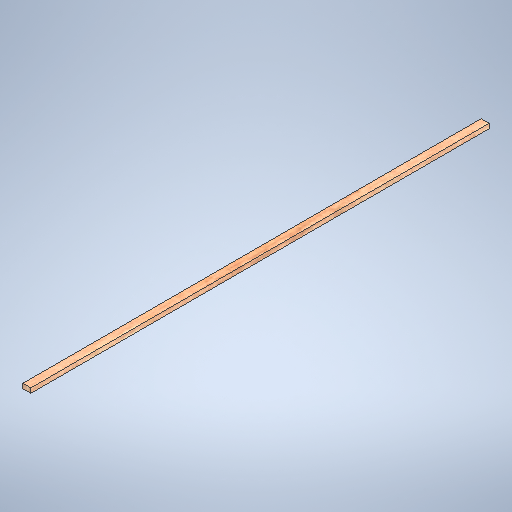
# Autodesk Inventor part: 2P.03.01.14.IM.AilTopSpanBeam
Saved by Autodesk Inventor 2025.2 (Build 292293000, 293)
## iProperties
Created: 2025-01-08
Part Number: 2P.03.01.14.IM.AilTopSpanBeam
Material: Wood (Birch)
Document SubType Name: Modeling
Designer: Imist
Density: 0.55 g/cm^3
Appearance: Birch - Natural Polished
Author: Imist
Autodesk Inventor part; units mm, degrees
ref_plane "YZ Plane" through (0, 0, 0) normal (1, 0, 0) x (0, 1, 0)
ref_plane "XZ Plane" through (0, 0, 0) normal (0, 1, 0) x (-1, 0, 0)
ref_plane "XY Plane" through (0, 0, 0) normal (0, 0, 1) x (1, 0, 0)
sketch "Sketch1" plane through (0, 0, 0) normal (0, 0, 1) x (1, 0, 0)
  line L0 (-2.548, 1.5) -> (2.548, 1.5)
  line L1 (2.548, 1.5) -> (2.548, -1.5)
  line L2 (2.548, -1.5) -> (-2.548, -1.5)
  line L3 (-2.548, -1.5) -> (-2.548, 1.5)
  line L4 (-2.548, 1.5) -> (2.548, -1.5) construction
  line L5 (2.548, 1.5) -> (-2.548, -1.5) construction
  point P0 (0, 0)
  point P1 (0, 0)
  dimension "d0" = 5.096
  dimension "d1" = 3
  constraints: 12 end point, 2 coincident, 2 midpoint, 2 parallel, 1 horizontal, 1 perpendicular
  measures "d0" distance of L1.end L2.end
  measures "d1" distance of L0.end L1.end
extrude "Extrusion1" add sketch "Sketch1" along normal blind 293
body "Solid1"
